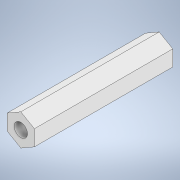
# Autodesk Inventor part: Spacer-M3H28
Saved by Autodesk Inventor 2022 (Build 260153000, 153)
## iProperties
Created: 2024-07-01
Part Number: Spacer-M3H28
Material: 一般
Document SubType Name: Modeling
Designer: yamashita1
Density: 1 g/cm^3
Appearance: 滑らか - 白
Author: yamashita1
Autodesk Inventor part; units mm, degrees
ref_plane "YZ Plane" through (0, 0, 0) normal (1, 0, 0) x (0, 1, 0)
ref_plane "XZ Plane" through (0, 0, 0) normal (0, 1, 0) x (-1, 0, 0)
ref_plane "XY Plane" through (0, 0, 0) normal (0, 0, 1) x (1, 0, 0)
sketch "スケッチ1" plane through (0, 0, 0) normal (0, 0, 1) x (1, 0, 0)
  line L0 (2.75, -1.5877) -> (0, -3.1754)
  line L1 (0, -3.1754) -> (-2.75, -1.5877)
  line L2 (-2.75, -1.5877) -> (-2.75, 1.5877)
  line L3 (-2.75, 1.5877) -> (0, 3.1754)
  line L4 (0, 3.1754) -> (2.75, 1.5877)
  line L5 (2.75, 1.5877) -> (2.75, -1.5877)
  circle A0 centre (0, 0) radius 1.35
  dimension "d0" = 5.5
  dimension "d1" = 2.7
  constraints: 12 end point, 2 coincident, 1 centre point, 1 vertical alignment, 13 other
  measures "d0" distance between parallel lines of L5 L2
  measures "d1" diameter of A0
extrude "押し出し1" add sketch "スケッチ1" along normal blind 28
